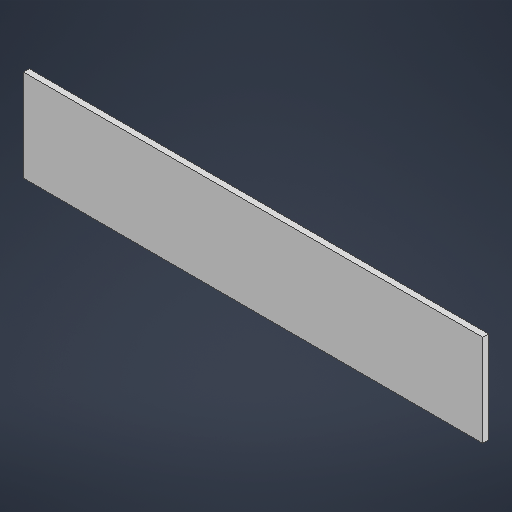
# Autodesk Inventor part: Pedalbox_V2_Vert_Rectangle
Saved by Autodesk Inventor 2026.1 (Build 301233000, 233)
## iProperties
Created: 2026-09-15
Part Number: Pedalbox_V2_Vert_Rectangle
Material: Generic
Document SubType Name: Modeling
Designer: share
Density: 1 g/cm^3
Appearance: Default
Author: share
Autodesk Inventor part; units mm, degrees
ref_plane "YZ Plane" through (0, 0, 0) normal (1, 0, 0) x (0, 1, 0)
ref_plane "XZ Plane" through (0, 0, 0) normal (0, 1, 0) x (-1, 0, 0)
ref_plane "XY Plane" through (0, 0, 0) normal (0, 0, 1) x (1, 0, 0)
sketch "Sketch1" plane through (0, 0, 0) normal (0, 0, 1) x (1, 0, 0)
  line L0 (125, -25) -> (-125, -25)
  line L1 (-125, -25) -> (-125, 25)
  line L2 (-125, 25) -> (125, 25)
  line L3 (125, 25) -> (125, -25)
  line L4 (0, 35) -> (0, -35) construction
  line L5 (-175, 0) -> (175, 0) construction
  point P0 (0, 0)
  dimension "d0" = 250
  dimension "d1" = 50
  constraints: 8 end point, 2 parallel, 1 horizontal, 1 perpendicular, 2 other
  measures "d0" distance between parallel lines of L3 L1
  measures "d1" distance between parallel lines of L0 L2
extrude "Extrusion1" add sketch "Sketch1" along normal mid plane 3.175
body "Solid1"
